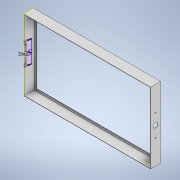
# Autodesk Inventor part: marco_ir
Saved by Autodesk Inventor 2021 (Build 250183000, 183)
## iProperties
Created: 2021-11-08
Part Number: marco_ir
Material: Genérico
Document SubType Name: Modeling
Designer: arthu
Density: 1 g/cm^3
Appearance: Valor por defecto
Author: arthu
Autodesk Inventor part; units mm, degrees
ref_plane "YZ Plane" through (0, 0, 0) normal (1, 0, 0) x (0, 1, 0)
ref_plane "XZ Plane" through (0, 0, 0) normal (0, 1, 0) x (-1, 0, 0)
ref_plane "XY Plane" through (0, 0, 0) normal (0, 0, 1) x (1, 0, 0)
sketch "Boceto1" plane through (0, 0, 0) normal (0, 0, 1) x (1, 0, 0)
  line L0 (261.2, -146.2) -> (-261.2, -146.2)
  line L1 (-261.2, -146.2) -> (-261.2, 146.2)
  line L2 (-261.2, 146.2) -> (261.2, 146.2)
  line L3 (261.2, 146.2) -> (261.2, -146.2)
  line L4 (261.2, -146.2) -> (-261.2, 146.2) construction
  line L5 (-261.2, -146.2) -> (261.2, 146.2) construction
  line L6 (250, -135) -> (-250, -135)
  line L7 (-250, -135) -> (-250, 135)
  line L8 (-250, 135) -> (250, 135)
  line L9 (250, 135) -> (250, -135)
  line L10 (250, -135) -> (-250, 135) construction
  line L11 (-250, -135) -> (250, 135) construction
  point P0 (0, 0)
  dimension "d0" = 522.4
  dimension "d1" = 292.4
  dimension "d2" = 500
  dimension "d3" = 270
  constraints: 24 end point, 4 midpoint, 4 parallel, 2 horizontal, 2 perpendicular
  measures "d0" distance of L1.end L2.end
  measures "d1" distance of L0.end L1.end
  measures "d2" distance of L7.end L8.end
  measures "d3" distance of L6.end L7.end
extrude "Extrusión1" add sketch "Boceto1" along normal blind 1.2
sketch "Boceto2" plane through (0, 0, 1.2) normal (0, 0, 1) x (1, 0, 0)
  line L0 (261.2, 146.2) -> (-261.2, 146.2) projected
  line L1 (-261.2, 146.2) -> (-261.2, -146.2) projected
  line L2 (261.2, -146.2) -> (261.2, 146.2) projected
  line L3 (-261.2, -146.2) -> (261.2, -146.2) projected
  line L4 (-260, 145) -> (260, 145)
  line L5 (260, 145) -> (260, -145)
  line L6 (260, -145) -> (-260, -145)
  line L7 (-260, -145) -> (-260, 145)
  point P0 (0, 0)
  dimension "d6" = 1.2
  constraints: 8 end point, 3 other
  measures "d6" distance between parallel lines of L0 L4
extrude "Extrusión2" add sketch "Boceto2" along normal blind 40
sketch "Boceto3" plane through (-261.2, -146.2, 0) normal (-1, 0, 0) x (0, 0, 1)
  line L0 (41.2, 292.4) -> (41.2, 0) projected
  line L1 (0, 292.4) -> (0, 0) projected
  line L2 (0, 0) -> (41.2, 0) projected
  line L3 (41.2, 292.4) -> (41.2, 0) projected
  line L4 (0, 292.4) -> (41.2, 292.4) projected
  circle A0 centre (20.6, 146.2) radius 10
  line L5 (10.6, 191.2) -> (30.6, 191.2)
  line L6 (30.6, 191.2) -> (30.6, 101.2)
  line L7 (30.6, 101.2) -> (10.6, 101.2)
  line L8 (10.6, 101.2) -> (10.6, 191.2)
  line L9 (10.6, 191.2) -> (30.6, 101.2) construction
  line L10 (30.6, 191.2) -> (10.6, 101.2) construction
  circle A1 centre (20.6, 191.2) radius 2.5
  circle A2 centre (20.6, 101.2) radius 2.5
  point P0 (0, 146.2)
  dimension "d9" = 20
  dimension "d12" = 90
  dimension "d13" = 5
  dimension "d14" = 5
  constraints: 12 end point, 4 midpoint, 3 centre point, 2 parallel, 1 horizontal, 1 perpendicular
  measures "d9" diameter of A0
  measures "d12" distance of L5.end L6.end
  measures "d13" diameter of A1
  measures "d14" diameter of A2
extrude "Extrusión3" cut sketch "Boceto3" against normal blind 1000 contours A0
extrude "Extrusión4" cut sketch "Boceto3" against normal blind 1000 contours A1 L5 | L5 A1 | A2 L7 | L7 A2
